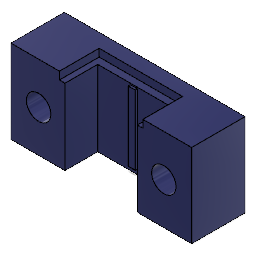
1-plug-mount Small v1 v1 (Autodesk Fusion 360 design; units mm, degrees)
Autodesk Fusion 360 part; units mm, degrees
sketch "Sketch1" plane through (0, 0, 0) normal (0, 0, 1) x (1, 0, 0) in component "PlugMountSmall"
  line L0 (-13, 25.63) -> (13, 25.63)
  line L1 (13, 25.63) -> (13, 13.63)
  line L2 (13, 13.63) -> (-13, 13.63)
  line L3 (-13, 13.63) -> (-13, 25.63)
  line L4 (0, 25.63) -> (0, 13.63) construction
  line L5 (13, 19.63) -> (-13, 19.63) construction
  line L6 (-0.5, 24.33) -> (0.5, 24.33)
  line L7 (0.5, 24.33) -> (0.5, 14.33)
  line L8 (0.5, 14.33) -> (-0.5, 14.33)
  line L9 (-0.5, 14.33) -> (-0.5, 24.33)
  line L10 (-6, 25.63) -> (-6, 24.53)
  line L11 (-6, 24.53) -> (-5.2, 24.53)
  line L12 (-5.2, 24.53) -> (-5.2, 13.63)
  circle A0 centre (-9, 19.63) radius 1.75
  circle A1 centre (9, 19.63) radius 1.75
  line L13 (5.2, 24.53) -> (5.2, 13.63)
  line L14 (6, 24.53) -> (5.2, 24.53)
  line L15 (6, 25.63) -> (6, 24.53)
  line L16 (-5.2, 24.53) -> (5.2, 24.53)
  dimension "d44_1" = 26
  dimension "d45_1" = 12
  dimension "d46_1" = 10
  dimension "d47_1" = 1.3
  dimension "d48_1" = 1
  dimension "d49_1" = 0.5
  dimension "d50_1" = 3.5
  dimension "d51_1" = 0.8
  dimension "d52_1" = 1.1
  dimension "d53_1" = 7
  dimension "d54_1" = 4
  constraint horizontal L0
  constraint vertical L1
  constraint horizontal L2
  constraint vertical L3
  constraint midpoint L0 L4.start
  constraint midpoint L2 L4.end
  constraint midpoint L1 L5.start
  constraint midpoint L3 L5.end
  constraint horizontal L6
  constraint vertical L7
  constraint horizontal L8
  constraint vertical L9
  constraint coincident L0 L10.start
  constraint perpendicular L0 L10
  constraint perpendicular L10 L11
  constraint coincident L2 L12.end
  constraint perpendicular L2 L12
  constraint coincident L5 A0.centre
  constraint symmetric L4 L10.start L15.start
  constraint symmetric L4 L10.end L14.start
  constraint symmetric L4 L11.end L13.start
  constraint symmetric L4 L12.end L13.end
  constraint symmetric L4 A0 A1
  measures "d44_1" distance of L0.start L0.end
  measures "d45_1" distance of L0.end L1.end
  measures "d46_1" distance of L6.end L7.end
  measures "d47_1" distance of L0 L6
  measures "d48_1" distance of L6.start L6.end
  measures "d49_1" distance of L4 L7
  measures "d50_1" diameter of A0
  measures "d51_1" distance of L10.end L11.end
  measures "d52_1" distance of L10.start L10.end
  measures "d53_1" distance of L3 L10
  measures "d54_1" distance of L5.end A0.centre
extrude "Extrude1" add sketch "Sketch1" along normal blind 3 contours L2 L12 L13 L16 | L6 L7 L8 L9 in component "PlugMountSmall"
extrude "Extrude2" add sketch "Sketch1" along normal blind 3.3 contours L6 L7 L8 L9 in component "PlugMountSmall"
extrude "Extrude3" add sketch "Sketch1" along normal blind 2 contours L0 L10 L11 L14 L15 L16 in component "PlugMountSmall"
extrude "Extrude4" add sketch "Sketch1" along normal blind 7.7 contours L0 L2 L3 L10 L11 L12 | L0 L1 L2 L13 L14 L15 in component "PlugMountSmall"
component "PlugMountSmall" placed x (1, 0, 0) y (0, 1, 0) z (0, 0, 1) at (0, 0, 0)
